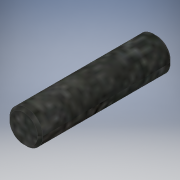
# Autodesk Inventor part: 1_4X1_DOWEL_PIN
Saved by Autodesk Inventor 2019.4 (Build 234330000, 330)
## iProperties
Created: 2020-02-01
Part Number: 1_4X1_DOWEL_PIN
Material: Steel
Document SubType Name: Modeling
Designer: mavericks
Density: 7.85 g/cm^3
Appearance: Plate
Author: mavericks
Autodesk Inventor part; units mm, degrees
ref_plane "YZ Plane" through (0, 0, 0) normal (1, 0, 0) x (0, 1, 0)
ref_plane "XZ Plane" through (0, 0, 0) normal (0, 1, 0) x (-1, 0, 0)
ref_plane "XY Plane" through (0, 0, 0) normal (0, 0, 1) x (1, 0, 0)
sketch "Sketch1" plane through (0, 0, 0) normal (0, 0, 1) x (1, 0, 0)
  circle A0 centre (0, 0) radius 3.175
  dimension "d0" = 6.35
  constraints: 1 centre point, 1 coincident
  measures "d0" diameter of A0
extrude "Extrusion1" add sketch "Sketch1" along normal mid plane 25.4
chamfer "Chamfer1" distance 0.508 angle 45 2 edges at (-3.175, 0, 12.7) (-3.175, 0, -12.7)
body "Solid1"
